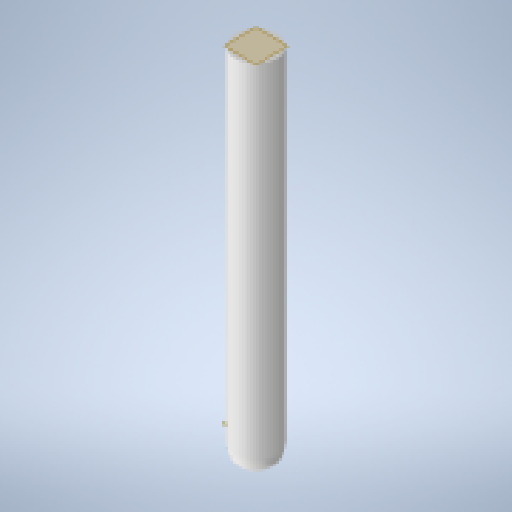
# Autodesk Inventor part: ForearmActuatorBodyBoundingBoxReal
Saved by Autodesk Inventor 2023 (Build 270158000, 158)
## iProperties
Created: 2023-03-25
Part Number: ForearmActuatorBodyBoundingBoxReal
Material: Generic
Document SubType Name: Modeling
Designer: Val
Density: 1 g/cm^3
Appearance: Default
Author: Val
Autodesk Inventor part; units mm, degrees
ref_plane "YZ Plane" through (0, 0, 0) normal (1, 0, 0) x (0, 1, 0)
ref_plane "XZ Plane" through (0, 0, 0) normal (0, 1, 0) x (-1, 0, 0)
ref_plane "XY Plane" through (0, 0, 0) normal (0, 0, 1) x (1, 0, 0)
ref_plane "Work Plane2" through (0, 209.702, 0) normal (0, 1, 0) x (1, 0, 0)
ref_plane "Work Plane3" through (-24.7004, 7, 34.125) normal (0, -1, 0) x (-1, 0, 0)
sketch "Sketch3" plane through (-24.7004, 7, 34.125) normal (0, -1, 0) x (-1, 0, 0)
  circle A0 centre (-24.7004, 34.125) radius 13
  arc A1 (-14.7004, 42.4316) -> (-34.7004, 42.4316) centre (-24.7004, 34.125) ccw construction
  constraints: 1 centre point, 1 coincident, 1 concentric
extrude "Extrusion2" add sketch "Sketch3" against normal up to surface (202.702 mm away)
sketch "Sketch5" plane through (0, 0, 0) normal (1, 0, 0) x (0, 1, 0)
  arc A0 (-8.5144, 9.8237) -> (0, -13) centre (0, 0) ccw construction
  line L0 (7, 13) -> (7, -13) construction
  arc A1 (-13, 0) -> (0, -13) centre (0, 0) ccw
  line L1 (0, 0) -> (-16.2632, 0) construction
  line L2 (0, -13) -> (7, -13)
  line L3 (-13, 0) -> (7, 0)
  line L4 (7, -13) -> (7, 0)
  constraints: 8 end point, 5 point on circle, 2 centre point, 2 concentric, 2 horizontal, 1 collinear, 1 midpoint, 1 point on line, 3 other
revolve "Revolution1" add sketch "Sketch5" angle 360 about axis through (0, 0, 0) along (0, -1, 0)
body "Solid2"
